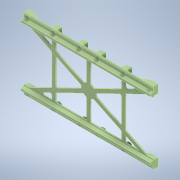
# Autodesk Inventor part: BodyStructure Centre
Saved by Autodesk Inventor 2022.2 (Build 262287000, 287)
## iProperties
Created: 2019-11-07
Part Number: BodyStructure Centre
Material: solidworks materials|ABS
Document SubType Name: Modeling
Designer: Jochen
Density: 1.02 g/cm^3
Appearance: 151,157,178
Sending System: SolidWorks 2017
Last Author: Felix
Last Saved: 2021-02-23
Author: Jochen
Autodesk Inventor part; units mm, degrees
ref_plane "YZ Plane" through (0, 0, 0) normal (1, 0, 0) x (0, 1, 0)
ref_plane "XZ Plane" through (0, 0, 0) normal (0, 1, 0) x (-1, 0, 0)
ref_plane "Work Plane1" through (0, 0, 30) normal (0, 0, 1) x (1, 0, 0)
sketch "Sketch1" plane through (0, 0, 30) normal (0, 0, 1) x (1, 0, 0)
  line L0 (-90, -50) -> (90, -50)
  line L1 (90, 50) -> (-90, 50)
  line L2 (90, 37) -> (82, 37)
  line L3 (0, -70) -> (0, 70) construction
  line L4 (-126, 0) -> (126, 0) construction
  line L5 (-51, -37) -> (-51, -27.519)
  line L6 (-46, -25.0935) -> (-46, -37)
  line L7 (-51, -27.519) -> (-70.5442, -37)
  line L8 (-82, -37) -> (-51, -21.9617)
  line L9 (51, -27.519) -> (70.5442, -37)
  line L10 (51, -37) -> (51, -27.519)
  line L11 (46, -25.0935) -> (46, -37)
  line L12 (82, -37) -> (51, -21.9617)
  line L13 (51, 27.519) -> (70.5442, 37)
  line L14 (82, 37) -> (51, 21.9617)
  line L15 (46, 37) -> (46, 25.0935)
  line L16 (46, 19.5362) -> (46, -19.5362)
  line L17 (51, -21.9617) -> (51, 21.9617)
  line L18 (51, 27.519) -> (51, 37)
  line L19 (-46, 37) -> (-46, 25.0935)
  line L20 (-46, 19.5362) -> (-46, -19.5362)
  line L21 (-51, -21.9617) -> (-51, 21.9617)
  line L22 (-46, 25.0935) -> (-46, 37)
  line L23 (-82, 37) -> (-51, 21.9617)
  line L24 (-51, 27.519) -> (-70.5442, 37)
  line L25 (-46, 19.5362) -> (-5.7279, 0)
  line L26 (2.5, -3.9914) -> (46, -25.0935)
  line L27 (-46, -19.5362) -> (-5.7279, 0)
  line L28 (2.5, 3.9914) -> (46, 25.0935)
  line L29 (46, 19.5362) -> (5.7279, 0)
  line L30 (-2.5, -3.9914) -> (-46, -25.0935)
  line L31 (46, -19.5362) -> (5.7279, 0)
  line L32 (-2.5, 3.9914) -> (-46, 25.0935)
  line L33 (-90, 37) -> (-82, 37)
  line L34 (-51, 27.519) -> (-51, 37)
  line L35 (70.5442, 37) -> (51, 37)
  line L36 (-70.5442, 37) -> (-51, 37)
  line L37 (-46, 37) -> (46, 37)
  line L38 (-82, -37) -> (-90, -37)
  line L39 (-51, -37) -> (-70.5442, -37)
  line L40 (46, -37) -> (-46, -37)
  line L41 (90, -37) -> (82, -37)
  line L42 (70.5442, -37) -> (51, -37)
  line L43 (90, -50) -> (90, -37)
  line L44 (90, 37) -> (90, 50)
  line L45 (-90, 50) -> (-90, 37)
  line L46 (-90, -37) -> (-90, -50)
  line L47 (-2.5, 37) -> (-2.5, 3.9914)
  line L48 (2.5, 37) -> (2.5, 3.9914)
  line L49 (2.5, -3.9914) -> (2.5, -37)
  line L50 (-2.5, -3.9914) -> (-2.5, -37)
  point P0 (0, 0)
  point P1 (-0.0551, -2.8054)
  point P2 (-0.0551, 2.8054)
  dimension "d1" = 5
  dimension "d2" = 5
  dimension "d3" = 8
  dimension "d4" = 180
  dimension "d5" = 13
  dimension "d7" = 100
  dimension "d8" = 46
  dimension "d12" = 5
  constraints: 99 end point, 39 parallel, 31 collinear, 14 perpendicular, 12 point on line, 9 horizontal, 3 vertical, 21 other
  measures "d1" distance between parallel lines of L8 L7
  measures "d2" distance between parallel lines of L6 L5
  measures "d3" distance of L8.start L38.end
  measures "d4" distance of L0.start L0.end
  measures "d5" distance of L38.end L0.start
  measures "d7" distance between parallel lines of L1 L0
  measures "d8" distance between parallel lines of L3 L6
  measures "d12" distance between parallel lines of L49 L50
extrude "Extrusion1" add sketch "Sketch1" along normal blind 12.5
fillet "Fillet1" radius 2 28 edges at (-51, -21.9617, 36.25) (-51, -37, 36.25) (-46, -37, 36.25) (-46, -19.5362, 36.25) (-46, -25.0935, 36.25) (-51, -27.519, 36.25) (-70.5442, -37, 36.25) (-51, 21.9617, 36.25) (-82, 37, 36.25) (-70.5442, 37, 36.25) (-51, 37, 36.25) (-51, 27.519, 36.25) (46, -25.0935, 36.25) (51, -27.519, 36.25) (51, -21.9617, 36.25) (46, -19.5362, 36.25) (46, -37, 36.25) (51, -37, 36.25) (46, 19.5362, 36.25) (51, 21.9617, 36.25) (51, 37, 36.25) (51, 27.519, 36.25) (70.5442, 37, 36.25) (-46, 19.5362, 36.25) (-46, 37, 36.25) (-46, 25.0935, 36.25) (46, 25.0935, 36.25) (46, 37, 36.25)
chamfer "Chamfer1" distance 5 angle 45 6 edges at (-5.7279, 0, 36.25) (-2.5, -3.9914, 36.25) (-2.5, 3.9914, 36.25) (2.5, 3.9914, 36.25) (5.7279, 0, 36.25) (2.5, -3.9914, 36.25)
fillet "Fillet2" radius 2 12 edges at (-6.9986, -6.1737, 36.25) (-2.5, -8.9914, 36.25) (-10.2265, -2.1823, 36.25) (-10.2265, 2.1823, 36.25) (-6.9986, 6.1737, 36.25) (-2.5, 8.9914, 36.25) (2.5, 8.9914, 36.25) (6.9986, 6.1737, 36.25) (10.2265, 2.1823, 36.25) (10.2265, -2.1823, 36.25) (6.9986, -6.1737, 36.25) (2.5, -8.9914, 36.25)
sketch "Sketch3" plane through (0, 0, 0) normal (1, 0, 0) x (0, 1, 0)
  line L0 (0, -8.5) -> (0, 51) construction
  line L1 (-70.5799, 0) -> (70.5799, 0) construction
  line L2 (-37, 42.5) -> (-50, 42.5) construction
  line L3 (-50, 42.5) -> (-37, 42.5) construction
  line L4 (-37, 42.5) -> (-22.5085, 42.5) construction
  line L5 (-20.709, 42.5) -> (-22.5085, 42.5) construction
  line L6 (-20.709, 42.5) -> (20.709, 42.5) construction
  line L7 (22.5085, 42.5) -> (20.709, 42.5) construction
  line L8 (22.5085, 42.5) -> (37, 42.5) construction
  line L9 (37, 42.5) -> (50, 42.5) construction
  line L10 (50, 42.5) -> (37, 42.5) construction
  line L11 (36.7994, 42.5) -> (37, 42.5) construction
  line L12 (36.7994, 42.5) -> (22.5085, 42.5) construction
  line L13 (20.709, 42.5) -> (22.5085, 42.5) construction
  line L14 (20.709, 42.5) -> (-20.709, 42.5) construction
  line L15 (-22.5085, 42.5) -> (-20.709, 42.5) construction
  line L16 (-22.5085, 42.5) -> (-37, 42.5) construction
  line L17 (-37, 42.5) -> (-10.0986, 42.5) construction
  line L18 (-8.4037, 42.5) -> (-10.0986, 42.5) construction
  line L19 (-6.7614, 42.5) -> (-8.4037, 42.5) construction
  line L20 (-6.657, 42.5) -> (-6.7614, 42.5) construction
  line L21 (-6.657, 42.5) -> (-24.5467, 42.5) construction
  line L22 (-26.3462, 42.5) -> (-24.5467, 42.5) construction
  line L23 (-26.3462, 42.5) -> (-35, 42.5) construction
  line L24 (-37, 42.5) -> (-35, 42.5) construction
  line L25 (37, 42.5) -> (10.0986, 42.5) construction
  line L26 (8.4037, 42.5) -> (10.0986, 42.5) construction
  line L27 (6.7614, 42.5) -> (8.4037, 42.5) construction
  line L28 (6.657, 42.5) -> (6.7614, 42.5) construction
  line L29 (6.657, 42.5) -> (24.5467, 42.5) construction
  line L30 (26.3462, 42.5) -> (24.5467, 42.5) construction
  line L31 (26.3462, 42.5) -> (35, 42.5) construction
  line L32 (37, 42.5) -> (35, 42.5) construction
  line L33 (28.9127, 42.5) -> (33.2006, 42.5) construction
  line L34 (37, 42.5) -> (33.2006, 42.5) construction
  line L35 (35, 42.5) -> (37, 42.5) construction
  line L36 (35, 42.5) -> (30.7121, 42.5) construction
  line L37 (28.9127, 42.5) -> (30.7121, 42.5) construction
  line L38 (18.1425, 42.5) -> (2.7291, 42.5) construction
  line L39 (0.9296, 42.5) -> (2.7291, 42.5) construction
  line L40 (-0.9296, 42.5) -> (0.9296, 42.5) construction
  line L41 (-2.7291, 42.5) -> (-0.9296, 42.5) construction
  line L42 (-2.7291, 42.5) -> (-18.1425, 42.5) construction
  line L43 (-16.3431, 42.5) -> (-18.1425, 42.5) construction
  line L44 (-16.3431, 42.5) -> (16.3431, 42.5) construction
  line L45 (18.1425, 42.5) -> (16.3431, 42.5) construction
  line L46 (16.3431, 42.5) -> (-16.3431, 42.5) construction
  line L47 (-18.1425, 42.5) -> (-16.3431, 42.5) construction
  line L48 (-18.1425, 42.5) -> (-2.7291, 42.5) construction
  line L49 (-0.9296, 42.5) -> (-2.7291, 42.5) construction
  line L50 (0.9296, 42.5) -> (-0.9296, 42.5) construction
  line L51 (2.7291, 42.5) -> (0.9296, 42.5) construction
  line L52 (2.7291, 42.5) -> (18.1425, 42.5) construction
  line L53 (16.3431, 42.5) -> (18.1425, 42.5) construction
  line L54 (30.7121, 42.5) -> (35, 42.5) construction
  line L55 (37, 42.5) -> (35, 42.5) construction
  line L56 (33.2006, 42.5) -> (37, 42.5) construction
  line L57 (33.2006, 42.5) -> (28.9127, 42.5) construction
  line L58 (30.7121, 42.5) -> (28.9127, 42.5) construction
  line L59 (-28.9127, 42.5) -> (-37, 42.5) construction
  line L60 (-35, 42.5) -> (-37, 42.5) construction
  line L61 (-35, 42.5) -> (-30.7121, 42.5) construction
  line L62 (-28.9127, 42.5) -> (-30.7121, 42.5) construction
  line L63 (-33.2006, 42.5) -> (-37, 42.5) construction
  line L64 (-33.2006, 42.5) -> (-28.9127, 42.5) construction
  line L65 (-30.7121, 42.5) -> (-28.9127, 42.5) construction
  line L66 (-30.7121, 42.5) -> (-35, 42.5) construction
  line L67 (-37, 42.5) -> (-35, 42.5) construction
  line L68 (35, 42.5) -> (37, 42.5) construction
  line L69 (35, 42.5) -> (26.3462, 42.5) construction
  line L70 (24.5467, 42.5) -> (26.3462, 42.5) construction
  line L71 (24.5467, 42.5) -> (6.657, 42.5) construction
  line L72 (6.7614, 42.5) -> (6.657, 42.5) construction
  line L73 (8.4037, 42.5) -> (6.7614, 42.5) construction
  line L74 (10.0986, 42.5) -> (8.4037, 42.5) construction
  line L75 (10.0986, 42.5) -> (37, 42.5) construction
  line L76 (-35, 42.5) -> (-37, 42.5) construction
  line L77 (-35, 42.5) -> (-26.3462, 42.5) construction
  line L78 (-24.5467, 42.5) -> (-26.3462, 42.5) construction
  line L79 (-24.5467, 42.5) -> (-6.657, 42.5) construction
  line L80 (-6.7614, 42.5) -> (-6.657, 42.5) construction
  line L81 (-8.4037, 42.5) -> (-6.7614, 42.5) construction
  line L82 (-10.0986, 42.5) -> (-8.4037, 42.5) construction
  line L83 (-10.0986, 42.5) -> (-37, 42.5) construction
  line L84 (-37, 30) -> (-50, 30) construction
  line L85 (-22.5085, 30) -> (-37, 30) construction
  line L86 (-20.709, 30) -> (-22.5085, 30) construction
  line L87 (20.709, 30) -> (-20.709, 30) construction
  line L88 (22.5085, 30) -> (20.709, 30) construction
  line L89 (36.7994, 30) -> (22.5085, 30) construction
  line L90 (37, 30) -> (36.7994, 30) construction
  line L91 (50, 30) -> (37, 30) construction
  line L92 (37, 30) -> (50, 30) construction
  line L93 (22.5085, 30) -> (37, 30) construction
  line L94 (20.709, 30) -> (22.5085, 30) construction
  line L95 (-20.709, 30) -> (20.709, 30) construction
  line L96 (-22.5085, 30) -> (-20.709, 30) construction
  line L97 (-37, 30) -> (-22.5085, 30) construction
  line L98 (-50, 30) -> (-37, 30) construction
  line L99 (-37, 30) -> (-10.0986, 30) construction
  line L100 (-35, 30) -> (-37, 30) construction
  line L101 (-26.3462, 30) -> (-35, 30) construction
  line L102 (-24.5467, 30) -> (-26.3462, 30) construction
  line L103 (-6.657, 30) -> (-24.5467, 30) construction
  line L104 (-6.7614, 30) -> (-6.657, 30) construction
  line L105 (-8.4037, 30) -> (-6.7614, 30) construction
  line L106 (-10.0986, 30) -> (-8.4037, 30) construction
  line L107 (37, 30) -> (10.0986, 30) construction
  line L108 (35, 30) -> (37, 30) construction
  line L109 (26.3462, 30) -> (35, 30) construction
  line L110 (24.5467, 30) -> (26.3462, 30) construction
  line L111 (6.657, 30) -> (24.5467, 30) construction
  line L112 (6.7614, 30) -> (6.657, 30) construction
  line L113 (8.4037, 30) -> (6.7614, 30) construction
  line L114 (10.0986, 30) -> (8.4037, 30) construction
  line L115 (30.7121, 30) -> (28.9127, 30) construction
  line L116 (35, 30) -> (30.7121, 30) construction
  line L117 (37, 30) -> (35, 30) construction
  line L118 (33.2006, 30) -> (37, 30) construction
  line L119 (28.9127, 30) -> (33.2006, 30) construction
  line L120 (16.3431, 30) -> (18.1425, 30) construction
  line L121 (-16.3431, 30) -> (16.3431, 30) construction
  line L122 (-18.1425, 30) -> (-16.3431, 30) construction
  line L123 (-2.7291, 30) -> (-18.1425, 30) construction
  line L124 (-0.9296, 30) -> (-2.7291, 30) construction
  line L125 (0.9296, 30) -> (-0.9296, 30) construction
  line L126 (2.7291, 30) -> (0.9296, 30) construction
  line L127 (18.1425, 30) -> (2.7291, 30) construction
  line L128 (18.1425, 30) -> (16.3431, 30) construction
  line L129 (2.7291, 30) -> (18.1425, 30) construction
  line L130 (0.9296, 30) -> (2.7291, 30) construction
  line L131 (-0.9296, 30) -> (0.9296, 30) construction
  line L132 (-2.7291, 30) -> (-0.9296, 30) construction
  line L133 (-18.1425, 30) -> (-2.7291, 30) construction
  line L134 (-16.3431, 30) -> (-18.1425, 30) construction
  line L135 (16.3431, 30) -> (-16.3431, 30) construction
  line L136 (28.9127, 30) -> (30.7121, 30) construction
  line L137 (33.2006, 30) -> (28.9127, 30) construction
  line L138 (37, 30) -> (33.2006, 30) construction
  line L139 (35, 30) -> (37, 30) construction
  line L140 (30.7121, 30) -> (35, 30) construction
  line L141 (-30.7121, 30) -> (-28.9127, 30) construction
  line L142 (-35, 30) -> (-30.7121, 30) construction
  line L143 (-37, 30) -> (-35, 30) construction
  line L144 (-28.9127, 30) -> (-37, 30) construction
  line L145 (-35, 30) -> (-37, 30) construction
  line L146 (-30.7121, 30) -> (-35, 30) construction
  line L147 (-28.9127, 30) -> (-30.7121, 30) construction
  line L148 (-33.2006, 30) -> (-28.9127, 30) construction
  line L149 (-37, 30) -> (-33.2006, 30) construction
  line L150 (10.0986, 30) -> (37, 30) construction
  line L151 (8.4037, 30) -> (10.0986, 30) construction
  line L152 (6.7614, 30) -> (8.4037, 30) construction
  line L153 (6.657, 30) -> (6.7614, 30) construction
  line L154 (24.5467, 30) -> (6.657, 30) construction
  line L155 (26.3462, 30) -> (24.5467, 30) construction
  line L156 (35, 30) -> (26.3462, 30) construction
  line L157 (37, 30) -> (35, 30) construction
  line L158 (-10.0986, 30) -> (-37, 30) construction
  line L159 (-8.4037, 30) -> (-10.0986, 30) construction
  line L160 (-6.7614, 30) -> (-8.4037, 30) construction
  line L161 (-6.657, 30) -> (-6.7614, 30) construction
  line L162 (-24.5467, 30) -> (-6.657, 30) construction
  line L163 (-26.3462, 30) -> (-24.5467, 30) construction
  line L164 (-35, 30) -> (-26.3462, 30) construction
  line L165 (-37, 30) -> (-35, 30) construction
  line L166 (50, 30) -> (50, 42.5) construction
  line L167 (50, 30) -> (50, 42.5) construction
  line L168 (37, 30) -> (37, 42.5) construction
  line L169 (37, 30) -> (37, 42.5) construction
  line L170 (-50, 30) -> (-50, 42.5) construction
  line L171 (-50, 30) -> (-50, 42.5) construction
  line L172 (-37, 30) -> (-37, 42.5) construction
  line L173 (-37, 30) -> (-37, 42.5) construction
  line L174 (-50, 30) -> (-50, 36.5)
  line L175 (-48, 38.5) -> (-43.9559, 38.5)
  line L176 (-43.9559, 38.5) -> (-42.5, 42.5)
  line L177 (-42.5, 42.5) -> (-40, 42.5)
  line L178 (-40, 42.5) -> (-38.5441, 38.5)
  line L179 (-38.5441, 38.5) -> (38.5441, 38.5)
  line L180 (38.5441, 38.5) -> (40, 42.5)
  line L181 (40, 42.5) -> (42.5, 42.5)
  line L182 (42.5, 42.5) -> (43.9559, 38.5)
  line L183 (50, 36.5) -> (50, 30)
  line L184 (50, 30) -> (-50, 30)
  line L185 (-41.25, 42.5) -> (-41.25, 30) construction
  line L186 (48, 38.5) -> (43.9559, 38.5)
  arc A0 (-48, 38.5) -> (-50, 36.5) centre (-48, 36.5) ccw
  arc A1 (50, 36.5) -> (48, 38.5) centre (48, 36.5) ccw
  point P0 (0, 0)
  point P1 (-50, 33.25)
  point P2 (50, 33)
  point P3 (48, 35)
  dimension "d28" = 110
  dimension "d29" = 2.5
  dimension "d30" = 4
  dimension "d37" = 10
  dimension "d38" = 2
  constraints: 26 end point, 7 point on line, 4 point on circle, 4 tangent, 3 collinear, 3 parallel, 3 perpendicular, 2 centre point, 2 midpoint, 1 equal radius, 1 horizontal, 1 vertical, 4 other
  measures "d28" angle of L176 L177
  measures "d29" distance of L176.end L177.end
  measures "d30" distance between parallel lines of L175 L177
  measures "d37" distance from line of L170 L177.end
  measures "d38" radius of A0
extrude "Extrusion3" cut sketch "Sketch3" along normal through all both and the other way through all keep common part
sketch "Sketch5" plane through (0, 0, 0) normal (0, 1, 0) x (-1, 0, 0)
  line L0 (126, 0) -> (-126, 0) construction
  line L1 (0, -8.5) -> (0, 51) construction
  line L2 (90, 38.5) -> (90, 42.5) construction
  line L3 (90, 42.5) -> (-90, 42.5) construction
  line L4 (-90, 42.5) -> (-90, 38.5) construction
  line L5 (90, 38.5) -> (-90, 38.5) construction
  line L6 (-90, 30) -> (-90, 36.5) construction
  line L7 (-90, 30) -> (90, 30) construction
  line L8 (90, 30) -> (90, 36.5) construction
  line L9 (90, 36.5) -> (90, 38.5) construction
  line L10 (-90, 38.5) -> (-90, 36.5) construction
  line L11 (90, 36.5) -> (-90, 36.5) construction
  line L12 (-81, 31.5) -> (-71.4737, 37)
  line L13 (-71.4737, 37) -> (-52, 37)
  line L14 (-52, 37) -> (-52, 30)
  line L15 (-52, 30) -> (-45, 30)
  line L16 (-45, 30) -> (-45, 37)
  line L17 (-45, 37) -> (-16, 37)
  line L18 (-16, 37) -> (-16, 30)
  line L19 (-16, 30) -> (-9, 30)
  line L20 (-9, 30) -> (-9, 37)
  line L21 (-9, 37) -> (9, 37)
  line L22 (9, 37) -> (9, 30)
  line L23 (9, 30) -> (16, 30)
  line L24 (16, 30) -> (16, 37)
  line L25 (16, 37) -> (45, 37)
  line L26 (45, 37) -> (45, 30)
  line L27 (45, 30) -> (52, 30)
  line L28 (52, 30) -> (52, 37)
  line L29 (52, 37) -> (71.4737, 37)
  line L30 (71.4737, 37) -> (81, 31.5)
  line L31 (90, 31.5) -> (90, 42.5)
  line L32 (90, 30) -> (-90, 30) construction
  line L33 (90, 42.5) -> (-90, 42.5)
  line L34 (-90, 42.5) -> (-90, 31.5)
  line L35 (90, 38.5) -> (-90, 38.5) projected
  line L36 (90, 36.5) -> (-90, 36.5) projected
  line L37 (81, 31.5) -> (90, 31.5)
  line L38 (-90, 30) -> (-90, 38.5) projected
  line L39 (-90, 31.5) -> (-81, 31.5)
  point P0 (0, 0)
  point P1 (61.7369, 37)
  dimension "d44" = 30
  dimension "d46" = 38
  dimension "d47" = 7
  dimension "d48" = 9
  dimension "d49" = 5.5
  dimension "d50" = 12.5
  dimension "d51" = 11
  dimension "d52" = 9
  constraints: 48 end point, 15 point on line, 11 perpendicular, 4 collinear, 3 parallel, 1 midpoint, 4 other
  measures "d44" angle of L7 L30
  measures "d46" distance from line of L2.end L28
  measures "d47" distance between parallel lines of L28 L26
  measures "d48" distance between parallel lines of L1 L22
  measures "d49" distance from line of L3 point (61.737, 37)
  measures "d50" vertical distance of L27.end L2.end
  measures "d51" distance from line of L37 L2.end
  measures "d52" distance of L30.end L31.start
extrude "Extrusion5" cut sketch "Sketch5" along normal through all both and the other way through all contours L39 L34 L36 L12 | L36 L34 L35 L31 L30 L29 L28 L26 L25 L24 L22 L21 L20 L18 L17 L16 L14 L13 L12 | L36 L16 L15 L14 | L34 L33 L31 L35 | L36 L20 L19 L18 | L31 L37 L30 L36 | L36 L24 L23 L22 | L28 L27 L26 L36 keep common part
sketch "Sketch6" plane through (0, 0, 0) normal (1, 0, 0) x (0, 1, 0)
  line L0 (0, -8.5) -> (0, 51) construction
  line L1 (-70.2702, 0) -> (70.2702, 0) construction
  line L2 (-40, 42.5) -> (-38.5441, 38.5) construction
  line L3 (-38.5441, 38.5) -> (38.5441, 38.5) construction
  line L4 (38.5441, 38.5) -> (40, 42.5) construction
  line L5 (40, 42.5) -> (42.5, 42.5) construction
  line L6 (42.5, 42.5) -> (43.9559, 38.5) construction
  line L7 (43.9559, 38.5) -> (48, 38.5) construction
  line L8 (-48, 38.5) -> (-43.9559, 38.5) construction
  line L9 (-43.9559, 38.5) -> (-42.5, 42.5) construction
  line L10 (-42.5, 42.5) -> (-40, 42.5) construction
  line L11 (-41.4365, 37) -> (-41.4365, 30)
  line L12 (-41.4365, 30) -> (41.4365, 30)
  line L13 (41.4365, 30) -> (41.4365, 37)
  line L14 (-50, 30) -> (-37, 30) construction
  line L15 (37, 30) -> (50, 30) construction
  line L16 (-41.4365, 37) -> (41.4365, 37)
  line L17 (37, 37) -> (49.9365, 37) projected
  arc A0 (49.9365, 37) -> (48, 38.5) centre (48, 36.5) ccw projected
  line L18 (49.9365, 37) -> (-49.9365, 37) projected
  arc A1 (-48, 38.5) -> (-49.9365, 37) centre (-48, 36.5) ccw projected
  point P0 (0, 0)
  point P1 (-49.9365, 35)
  point P2 (-41.4365, 33.5)
  point P3 (50, 35)
  dimension "d55" = 8.5
  dimension "d75" = 1.5
  constraints: 8 end point, 2 point on line, 1 horizontal, 1 midpoint, 1 vertical, 2 other
  measures "d55" horizontal distance of point (-41.436, 33.5) point (-49.936, 35)
  measures "d75" distance between parallel lines of L16 L3
extrude "Extrusion6" cut sketch "Sketch6" along normal mid plane 140
sketch "Sketch9" plane through (45, -49.9365, 37) normal (0, 0, -1) x (-1, 0, 0)
  arc A0 (-16.8391, 86.9365) -> (-17.712, 83.137) centre (-16.8391, 84.9365) ccw projected
  line L0 (-17.712, 83.137) -> (-8.8729, 78.8492) projected
  arc A1 (-8.8729, 78.8492) -> (-6, 80.6486) centre (-8, 80.6486) ccw projected
  arc A2 (-6, 84.9365) -> (-8, 86.9365) centre (-8, 84.9365) ccw projected
  line L1 (-8, 86.9365) -> (-16.8391, 86.9365) projected
  arc A3 (-6, 70.6455) -> (-7.1271, 72.445) centre (-8, 70.6455) ccw projected
  line L2 (-7.1271, 72.445) -> (-26.4737, 81.8301) projected
  line L3 (-26.4737, 99.873) -> (-26.4737, 81.8301) projected
  line L4 (-45, 86.9365) -> (-45, 99.873) projected
  line L5 (-37, 86.9365) -> (-45, 86.9365) projected
  line L6 (-26.4737, 81.8301) -> (-37, 86.9365) projected
  arc A4 (-7.1271, 27.428) -> (-6, 29.2274) centre (-8, 29.2274) ccw projected
  line L7 (-26.4737, 18.0428) -> (-7.1271, 27.428) projected
  line L8 (-45, 0) -> (-45, 12.9365) projected
  line L9 (-45, 12.9365) -> (-37, 12.9365) projected
  line L10 (-37, 12.9365) -> (-26.4737, 18.0428) projected
  line L11 (126.5866, 86.7359) -> (116.4737, 81.8301) projected
  arc A5 (127.4595, 86.9365) -> (126.5866, 86.7359) centre (127.4595, 84.9365) ccw projected
  line L12 (135, 86.9365) -> (127.4595, 86.9365) projected
  line L13 (135, 99.873) -> (135, 86.9365) projected
  line L14 (116.4737, 18.0428) -> (127, 12.9365) projected
  line L15 (127, 12.9365) -> (135, 12.9365) projected
  line L16 (135, 12.9365) -> (135, 0) projected
  arc A6 (-6, 19.2244) -> (-8.8729, 21.0238) centre (-8, 19.2244) ccw projected
  line L17 (-8.8729, 21.0238) -> (-25.5442, 12.9365) projected
  line L18 (-25.5442, 12.9365) -> (-8, 12.9365) projected
  arc A7 (-8, 12.9365) -> (-6, 14.9365) centre (-8, 14.9365) ccw projected
  circle A8 centre (-40, 94.9365) radius 1.5
  circle A9 centre (32.5, 94.9365) radius 1.5
  circle A10 centre (-3.5, 94.9365) radius 1.5
  circle A11 centre (57.5, 94.9365) radius 1.5
  circle A12 centre (93.5, 94.9365) radius 1.5
  circle A13 centre (130, 94.9365) radius 1.5
  circle A14 centre (130, 4.9365) radius 1.5
  circle A15 centre (93.5, 4.9365) radius 1.5
  circle A16 centre (57.5, 4.9365) radius 1.5
  circle A17 centre (-3.5, 4.9365) radius 1.5
  circle A18 centre (32.5, 4.9365) radius 1.5
  circle A19 centre (-40, 4.9365) radius 1.5
  line L19 (-40, 94.9365) -> (130, 94.9365) construction
  line L20 (130, 94.9365) -> (130, 4.9365) construction
  line L21 (130, 4.9365) -> (-40, 4.9365) construction
  line L22 (-40, 4.9365) -> (-40, 94.9365) construction
  line L23 (171, 49.9365) -> (-81, 49.9365) construction
  line L24 (45, -20.0635) -> (45, 119.9365) construction
  line L25 (32.5, 94.9365) -> (32.5, 4.9365) construction
  line L26 (-3.5, 4.9365) -> (-3.5, 94.9365) construction
  line L27 (93.5, 94.9365) -> (93.5, 4.9365) construction
  line L28 (135, 88.4806) -> (-45, 88.4806) construction
  line L29 (57.5, 94.9365) -> (57.5, 4.9365) construction
  circle A20 centre (-40, 4.9365) radius 2.9
  circle A21 centre (-3.5, 4.9365) radius 2.9
  circle A22 centre (32.5, 4.9365) radius 2.9
  circle A23 centre (57.5, 4.9365) radius 2.9
  circle A24 centre (93.5, 4.9365) radius 2.9
  circle A25 centre (130, 4.9365) radius 2.9
  circle A26 centre (130, 94.9365) radius 2.9
  circle A27 centre (93.5, 94.9365) radius 2.9
  circle A28 centre (57.5, 94.9365) radius 2.9
  circle A29 centre (32.5, 94.9365) radius 2.9
  circle A30 centre (-3.5, 94.9365) radius 2.9
  circle A31 centre (-40, 94.9365) radius 2.9
  arc A32 (48.4384, 41.5328) -> (47.5, 39.8379) centre (49.5, 39.8379) ccw projected
  line L30 (47.5, 39.8379) -> (47.5, 12.9365) projected
  line L31 (47.5, 12.9365) -> (89, 12.9365) projected
  arc A33 (89, 12.9365) -> (91, 14.9365) centre (89, 14.9365) ccw projected
  arc A34 (91, 23.5903) -> (89.8729, 25.3898) centre (89, 23.5903) ccw projected
  line L32 (89.8729, 25.3898) -> (52.9948, 43.2795) projected
  arc A35 (52.9948, 43.2795) -> (51.0603, 43.1751) centre (52.1219, 41.4801) ccw projected
  line L33 (51.0603, 43.1751) -> (48.4384, 41.5328) projected
  line L34 (54, 0) -> (54, 8.5) projected
  line L35 (61, 0) -> (54, 0) projected
  line L36 (90, 0) -> (90, 8.5) projected
  line L37 (90, 0) -> (61, 0) projected
  arc A36 (89.8729, 74.4832) -> (91, 76.2827) centre (89, 76.2827) ccw projected
  line L38 (52.9948, 56.5935) -> (89.8729, 74.4832) projected
  arc A37 (51.0603, 56.6979) -> (52.9948, 56.5935) centre (52.1219, 58.3929) ccw projected
  line L39 (48.4384, 58.3401) -> (51.0603, 56.6979) projected
  arc A38 (47.5, 60.0351) -> (48.4384, 58.3401) centre (49.5, 60.0351) ccw projected
  line L40 (47.5, 86.9365) -> (47.5, 60.0351) projected
  line L41 (54, 99.873) -> (61, 99.873) projected
  line L42 (61, 99.873) -> (61, 91.373) projected
  arc A39 (91, 84.9365) -> (89, 86.9365) centre (89, 84.9365) ccw projected
  line L43 (56.3536, 47.2074) -> (88.1271, 31.794) projected
  arc A40 (88.1271, 31.794) -> (91, 33.5934) centre (89, 33.5934) ccw projected
  line L44 (54, 0) -> (36, 0) projected
  line L45 (29, 0) -> (0, 0) projected
  arc A41 (0.1271, 25.3898) -> (-1, 23.5903) centre (1, 23.5903) ccw projected
  line L46 (1.8729, 31.794) -> (33.6464, 47.2074) projected
  arc A42 (-1, 33.5934) -> (1.8729, 31.794) centre (1, 33.5934) ccw projected
  arc A43 (1.8729, 68.079) -> (-1, 66.2796) centre (1, 66.2796) ccw projected
  line L47 (33.6464, 52.6655) -> (1.8729, 68.079) projected
  line L48 (97, 0) -> (90, 0) projected
  line L49 (116.4737, 0) -> (97, 0) projected
  line L50 (135, 0) -> (116.4737, 0) projected
  arc A44 (91, 66.2796) -> (88.1271, 68.079) centre (89, 66.2796) ccw projected
  line L51 (88.1271, 68.079) -> (56.3536, 52.6655) projected
  line L52 (36, 99.873) -> (54, 99.873) projected
  line L53 (36, 99.873) -> (36, 91.373) projected
  line L54 (29, 91.373) -> (29, 99.873) projected
  line L55 (0, 99.873) -> (29, 99.873) projected
  line L56 (0, 99.873) -> (0, 91.373) projected
  line L57 (61, 99.873) -> (90, 99.873) projected
  line L58 (36, 0) -> (29, 0) projected
  line L59 (42.5, 12.9365) -> (42.5, 39.8379) projected
  arc A45 (42.5, 39.8379) -> (41.5616, 41.5328) centre (40.5, 39.8379) ccw projected
  line L60 (41.5616, 41.5328) -> (38.9397, 43.1751) projected
  arc A46 (38.9397, 43.1751) -> (37.0052, 43.2795) centre (37.8781, 41.4801) ccw projected
  line L61 (37.0052, 43.2795) -> (0.1271, 25.3898) projected
  arc A47 (-1, 14.9365) -> (1, 12.9365) centre (1, 14.9365) ccw projected
  line L62 (0, 0) -> (-7, 0) projected
  line L63 (0.1271, 74.4832) -> (37.0052, 56.5935) projected
  arc A48 (-1, 76.2827) -> (0.1271, 74.4832) centre (1, 76.2827) ccw projected
  arc A49 (37.0052, 56.5935) -> (38.9397, 56.6979) centre (37.8781, 58.3929) ccw projected
  line L64 (38.9397, 56.6979) -> (41.5616, 58.3401) projected
  arc A50 (41.5616, 58.3401) -> (42.5, 60.0351) centre (40.5, 60.0351) ccw projected
  line L65 (42.5, 60.0351) -> (42.5, 86.9365) projected
  line L66 (42.5, 86.9365) -> (1, 86.9365) projected
  line L67 (97, 8.5) -> (97, 0) projected
  arc A51 (96, 29.2274) -> (97.1271, 27.428) centre (98, 29.2274) ccw projected
  line L68 (97.1271, 27.428) -> (116.4737, 18.0428) projected
  line L69 (29, 99.873) -> (36, 99.873) projected
  arc A52 (1, 86.9365) -> (-1, 84.9365) centre (1, 84.9365) ccw projected
  line L70 (-7, 99.873) -> (0, 99.873) projected
  line L71 (-7, 91.373) -> (-7, 99.873) projected
  line L72 (-45, 99.873) -> (-26.4737, 99.873) projected
  line L73 (90, 99.873) -> (97, 99.873) projected
  line L74 (97, 99.873) -> (116.4737, 99.873) projected
  line L75 (116.4737, 99.873) -> (135, 99.873) projected
  line L76 (116.4737, 81.8301) -> (116.4737, 99.873) projected
  line L77 (-7, 0) -> (-26.4737, 0) projected
  line L78 (-26.4737, 18.0428) -> (-26.4737, 0) projected
  line L79 (-26.4737, 0) -> (-45, 0) projected
  arc A53 (96, 14.9365) -> (98, 12.9365) centre (98, 14.9365) ccw projected
  line L80 (98, 12.9365) -> (106.8391, 12.9365) projected
  arc A54 (106.8391, 12.9365) -> (107.712, 16.7359) centre (106.8391, 14.9365) ccw projected
  line L81 (107.712, 16.7359) -> (98.8729, 21.0238) projected
  arc A55 (98.8729, 21.0238) -> (96, 19.2244) centre (98, 19.2244) ccw projected
  arc A56 (97.1271, 72.445) -> (96, 70.6455) centre (98, 70.6455) ccw projected
  line L82 (116.4737, 81.8301) -> (97.1271, 72.445) projected
  line L83 (-26.4737, 99.873) -> (-7, 99.873) projected
  arc A57 (98, 86.9365) -> (96, 84.9365) centre (98, 84.9365) ccw projected
  line L84 (106.8391, 86.9365) -> (98, 86.9365) projected
  arc A58 (107.712, 83.137) -> (106.8391, 86.9365) centre (106.8391, 84.9365) ccw projected
  line L85 (98.8729, 78.8492) -> (107.712, 83.137) projected
  arc A59 (96, 80.6486) -> (98.8729, 78.8492) centre (98, 80.6486) ccw projected
  line L86 (-1, 84.9365) -> (-1, 76.2827) projected
  line L87 (96, 19.2244) -> (96, 14.9365) projected
  line L88 (-1, 23.5903) -> (-1, 14.9365) projected
  line L89 (1, 12.9365) -> (42.5, 12.9365) projected
  line L90 (55.2265, 50.8661) -> (55.2265, 49.0069) projected
  arc A60 (55.2265, 49.0069) -> (56.3536, 47.2074) centre (57.2265, 49.0069) ccw projected
  line L91 (91, 33.5934) -> (91, 66.2796) projected
  arc A61 (56.3536, 52.6655) -> (55.2265, 50.8661) centre (57.2265, 50.8661) ccw projected
  line L92 (-6, 80.6486) -> (-6, 84.9365) projected
  line L93 (96, 84.9365) -> (96, 80.6486) projected
  line L94 (-6, 29.2274) -> (-6, 70.6455) projected
  line L95 (0, 91.373) -> (-7, 91.373) projected
  line L96 (36, 91.373) -> (29, 91.373) projected
  line L97 (54, 91.373) -> (54, 99.873) projected
  line L98 (61, 91.373) -> (54, 91.373) projected
  line L99 (90, 91.373) -> (90, 99.873) projected
  line L100 (97, 91.373) -> (90, 91.373) projected
  line L101 (97, 99.873) -> (97, 91.373) projected
  line L102 (-7, 0) -> (-7, 8.5) projected
  line L103 (-7, 8.5) -> (0, 8.5) projected
  line L104 (0, 8.5) -> (0, 0) projected
  line L105 (29, 0) -> (29, 8.5) projected
  line L106 (29, 8.5) -> (36, 8.5) projected
  line L107 (36, 8.5) -> (36, 0) projected
  line L108 (54, 8.5) -> (61, 8.5) projected
  line L109 (61, 8.5) -> (61, 0) projected
  line L110 (90, 8.5) -> (97, 8.5) projected
  line L111 (116.4737, 0) -> (116.4737, 18.0428) projected
  line L112 (96, 70.6455) -> (96, 29.2274) projected
  line L113 (-6, 14.9365) -> (-6, 19.2244) projected
  arc A62 (33.6464, 47.2074) -> (34.7735, 49.0069) centre (32.7735, 49.0069) ccw projected
  line L114 (34.7735, 49.0069) -> (34.7735, 50.8661) projected
  arc A63 (34.7735, 50.8661) -> (33.6464, 52.6655) centre (32.7735, 50.8661) ccw projected
  line L115 (-1, 66.2796) -> (-1, 33.5934) projected
  line L116 (91, 76.2827) -> (91, 84.9365) projected
  line L117 (89, 86.9365) -> (47.5, 86.9365) projected
  line L118 (91, 14.9365) -> (91, 23.5903) projected
  point P0 (45, 49.9365)
  dimension "d61" = 3
  dimension "d63" = 90
  dimension "d64" = 85
  dimension "d65" = 48.5
  dimension "d66" = 12.5
  dimension "d69" = 5.8
  constraints: 24 centre point, 22 equal radius, 16 end point, 15 coincident, 8 point on line, 4 perpendicular, 2 parallel, 1 horizontal, 4 other
  measures "d61" diameter of A8
  measures "d63" distance of L21.end L19.start
  measures "d64" distance from line of A19.centre L24
  measures "d65" distance from line of L26.start L24
  measures "d66" distance from line of L25.end L24
  measures "d69" diameter of A20
fillet "Fillet5" radius 3.5 17 edges at (-52, -41.4365, 33.5) (-45, -41.4365, 33.5) (-16, -41.4365, 33.5) (-9, -41.4365, 33.5) (0, -43.9559, 38.5) (9, -41.4365, 33.5) (16, -41.4365, 33.5) (45, -41.4365, 33.5) (52, -41.4365, 33.5) (52, 41.4365, 33.5) (45, 41.4365, 33.5) (16, 41.4365, 33.5) (9, 41.4365, 33.5) (-9, 41.4365, 33.5) (-16, 41.4365, 33.5) (-45, 41.4365, 33.5) (-52, 41.4365, 33.5)
fillet "Fillet4" radius 1 28 edges at (-12.5, -41.4365, 37) (-9, -47.4364, 37) (-16, -47.4364, 37) (9, -47.4364, 37) (12.5, -41.4365, 37) (16, -47.4364, 37) (52, -47.4364, 37) (48.5, -41.4365, 37) (45, -47.4364, 37) (-45, -47.4364, 37) (-48.5, -41.4365, 37) (-52, -47.4364, 37) (52, 47.4364, 37) (48.5, 41.4365, 37) (45, 47.4364, 37) (16, 47.4364, 37) (12.5, 41.4365, 37) (9, 47.4364, 37) (-9, 47.4364, 37) (-12.5, 41.4365, 37) (-16, 47.4364, 37) (-45, 47.4364, 37) (-48.5, 41.4365, 37) (-52, 47.4364, 37) (-71.4737, 40.9151, 37) (71.4737, 40.9151, 37) (71.4737, -40.9151, 37) (-71.4737, -40.9151, 37)
sketch "Sketch8" plane through (0, 0, 0) normal (0, 0, 1) x (1, 0, 0)
  line L0 (82, -37) -> (86.5505, -39.2075)
  line L1 (90, -40) -> (90, 40)
  line L2 (82, 37) -> (90, 37) projected
  line L3 (82, 37) -> (82, -37)
  line L4 (0, -70) -> (0, 70) construction
  line L5 (-126, 0) -> (126, 0) construction
  arc A0 (90, 40) -> (86.5505, 39.2075) centre (90, 32.0967) ccw
  line L6 (82, 37) -> (86.5505, 39.2075)
  arc A1 (86.5505, -39.2075) -> (90, -40) centre (90, -32.0967) ccw
  line L7 (81, -36.5149) -> (82, -37) projected
  line L8 (90, -37) -> (90, -50) projected
  line L9 (82, 37) -> (81, 36.5149) projected
  line L10 (81, 36.5149) -> (81, 50) projected
  line L11 (81, 50) -> (90, 50) projected
  line L12 (90, 50) -> (90, 37) projected
  line L13 (90, 37) -> (82, 37) projected
  line L14 (-82, -37) -> (-86.5505, -39.2075)
  line L15 (-90, -40) -> (-90, 40)
  line L16 (-82, 37) -> (-82, -37)
  line L17 (-82, 37) -> (-86.5505, 39.2075)
  arc A2 (-86.5505, 39.2075) -> (-90, 40) centre (-90, 32.0967) ccw
  arc A3 (-90, -40) -> (-86.5505, -39.2075) centre (-90, -32.0967) ccw
  point P0 (0, 0)
  constraints: 16 end point, 8 point on circle, 7 symmetric about line, 4 centre point, 4 tangent, 1 coincident, 1 collinear, 1 equal radius, 1 line through centre, 1 parallel, 1 point on line, 3 other
extrude "Extrusion7" [suppressed]
extrude "Extrusion8" cut sketch "Sketch9" along normal through all both and the other way through all contours A8 | A9 | A10 | A11 | A12 | A13 | A14 | A15 | A16 | A17 | A18 | A19
extrude "Extrusion9" cut sketch "Sketch9" along normal blind 1 and the other way blind 10 contours A8 | A9 | A10 | A11 | A12 | A13 | A14 | A15 | A16 | A17 | A18 | A19 | A20 | A21 | A22 | A23 | A24 | A25 | A26 | A27 | A28 | A29 | A30 | A31
sketch "Sketch10" plane through (0, 0, 0) normal (1, 0, 0) x (0, 1, 0)
  line L0 (-70.0019, 0) -> (70.0019, 0) construction
  line L1 (0, -8.5) -> (0, 51) construction
  line L2 (-38.5, 37) -> (38.5, 37)
  line L3 (38.5, 37) -> (38.5, 31.5)
  line L4 (38.5, 31.5) -> (-38.5, 31.5)
  line L5 (-38.5, 31.5) -> (-38.5, 37)
  line L6 (-31.7637, 37) -> (-49.9365, 37) construction
  line L7 (42.5, 42.5) -> (40, 42.5) construction
  line L8 (40.5, 42.5) -> (40.5, 31.5) construction
  line L9 (36.5149, 31.5) -> (50, 31.5) construction
  point P0 (0, 0)
  point P1 (-38.5441, 38.5)
  point P2 (38.5441, 38.5)
  dimension "d79" = 2
  dimension "d80" = 2
  constraints: 10 end point, 3 point on line, 2 parallel, 1 horizontal, 1 perpendicular, 1 vertical, 1 other
  measures "d79" distance of L7.start L8.start
  measures "d80" distance between parallel lines of L8 L3
extrude "Extrusion10" cut sketch "Sketch10" along normal through all both and the other way through all
equation "\"d2\" = d1"
equation "\"d12\" = d1"
body "Solid1"
body "Solid2"
